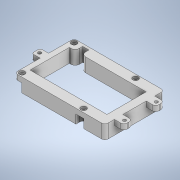
# Autodesk Inventor part: Pi3BatteryBoard_Mockup
Saved by Autodesk Inventor 2021 (Build 250183000, 183)
## iProperties
Created: 2021-04-19
Part Number: Pi3BatteryBoard_Mockup
Material: Generic
Document SubType Name: Modeling
Designer: trent
Density: 1 g/cm^3
Appearance: Default
Author: trent
Autodesk Inventor part; units mm, degrees
ref_plane "YZ Plane" through (0, 0, 0) normal (1, 0, 0) x (0, 1, 0)
ref_plane "XZ Plane" through (0, 0, 0) normal (0, 1, 0) x (-1, 0, 0)
ref_plane "XY Plane" through (0, 0, 0) normal (0, 0, 1) x (1, 0, 0)
sketch "Sketch1" plane through (0, 0, 0) normal (0, 1, 0) x (-1, 0, 0)
  line L0 (-3, 0) -> (-82, 0)
  line L1 (-85, -3) -> (-85, -53)
  line L2 (-82, -56) -> (-3, -56)
  line L3 (0, -53) -> (0, -3)
  arc A0 (-3, -56) -> (0, -53) centre (-3, -53) ccw
  arc A1 (0, -3) -> (-3, 0) centre (-3, -3) ccw
  arc A2 (-82, 0) -> (-85, -3) centre (-82, -3) ccw
  arc A3 (-85, -53) -> (-82, -56) centre (-82, -53) ccw
  circle A4 centre (-3.5, -52.5) radius 1.5
  circle A5 centre (-3.5, -3.5) radius 1.5
  circle A6 centre (-61.5, -52.5) radius 1.5
  circle A7 centre (-61.5, -3.5) radius 1.5
  point P0 (0, 0)
  point P1 (-85, -56)
  point P2 (-85, 0)
  point P3 (0, -56)
  dimension "d0" = 85
  dimension "d1" = 56
  dimension "d2" = 3
  dimension "d9" = 3
  dimension "d10" = 3
  dimension "d15" = 3
  dimension "d16" = 3
  dimension "d140" = 58
  dimension "d141" = 58
  dimension "d142" = 49
  dimension "d143" = 3.5
  constraints: 8 centre point, 8 end point, 8 point on circle, 8 point on line, 8 tangent, 3 equal radius, 2 parallel, 1 horizontal, 1 perpendicular
  measures "d0" distance of point (-85, -56) point (0, -56)
  measures "d1" distance of point (-85, 0) point (-85, -56)
  measures "d2" radius of A0
  measures "d9" diameter of A4
  measures "d10" diameter of A5
  measures "d15" diameter of A6
  measures "d16" diameter of A7
  measures "d140" distance of A6.centre A4.centre
  measures "d141" distance of A5.centre A7.centre
  measures "d142" distance of A4.centre A5.centre
  measures "d143" distance from line of L0 A5.centre
extrude "Extrusion1" add sketch "Sketch1" along normal blind 13
sketch "Sketch12" plane through (0, 0, 0) normal (0, -1, 0) x (1, 0, 0)
  line L0 (5, -9.5) -> (77.5, -9.5)
  line L1 (77.5, -9.5) -> (77.5, -46.5)
  line L2 (5, -46.5) -> (5, -9.5)
  line L3 (82, -56) -> (3, -56) projected
  line L4 (85, -3) -> (85, -53) projected
  line L5 (3, 0) -> (82, 0) projected
  line L6 (0, -53) -> (0, -3) projected
  line L7 (16.35, -50.5) -> (16.35, -53.65)
  line L8 (16.35, -53.65) -> (10.5, -53.65)
  line L9 (10.5, -53.65) -> (10.5, -50.5)
  line L10 (77.5, -46.5) -> (20.35, -46.5)
  line L11 (6.5, -46.5) -> (5, -46.5)
  arc A0 (10.5, -50.5) -> (6.5, -46.5) centre (6.5, -50.5) ccw
  arc A1 (20.35, -46.5) -> (16.35, -50.5) centre (20.35, -50.5) ccw
  point P0 (0, 0)
  point P1 (10.5, -46.5)
  point P2 (16.35, -46.5)
  dimension "d153" = 7.5
  dimension "d154" = 9.5
  dimension "d155" = 5
  dimension "d157" = 10.5
  dimension "d158" = 2.35
  dimension "d159" = 5.85
  dimension "d160" = 4
  constraints: 16 end point, 4 parallel, 4 point on circle, 4 point on line, 4 tangent, 2 centre point, 1 equal radius, 1 horizontal, 1 perpendicular
  measures "d153" distance between parallel lines of L4 L1
  measures "d154" distance between parallel lines of L5 L0
  measures "d155" distance between parallel lines of L6 L2
  measures "d157" distance between parallel lines of L6 L9
  measures "d158" distance between parallel lines of L3 L8
  measures "d159" distance of L7.end L8.end
  measures "d160" radius of A0
extrude "Extrusion12" cut sketch "Sketch12" against normal up to next
sketch "Sketch14" plane through (0, 13, 0) normal (0, 1, 0) x (1, 0, 0)
  circle A0 centre (3.5, 3.5) radius 1.5 projected
  circle A1 centre (3.5, 3.5) radius 2.625
  circle A2 centre (61.5, 3.5) radius 1.5 projected
  circle A3 centre (61.5, 3.5) radius 2.625
  circle A4 centre (61.5, 52.5) radius 1.5 projected
  circle A5 centre (61.5, 52.5) radius 2.625
  circle A6 centre (3.5, 52.5) radius 1.5 projected
  circle A7 centre (3.5, 52.5) radius 2.625
  point P0 (0, 0)
  dimension "d161" = 5.25
  dimension "d162" = 5.25
  dimension "d163" = 5.25
  dimension "d164" = 5.25
  constraints: 4 centre point, 4 coincident
  measures "d161" diameter of A1
  measures "d162" diameter of A7
  measures "d163" diameter of A5
  measures "d164" diameter of A3
extrude "Extrusion14" cut sketch "Sketch14" against normal blind 1.75 contours A0 | A1 | A2 | A3 | A4 | A5 | A6 | A7
sketch "Sketch15" plane through (0, 0, 0) normal (0, -1, 0) x (1, 0, 0)
  arc A0 (3.5, -6.75) -> (6.75, -3.5) centre (3.5, -3.5) ccw
  arc A1 (57.75, -3.5) -> (65.25, -3.5) centre (61.5, -3.5) ccw
  arc A2 (65.25, -52.5) -> (57.75, -52.5) centre (61.5, -52.5) ccw
  arc A3 (6.75, -52.5) -> (3.5, -49.25) centre (3.5, -52.5) ccw
  line L0 (57.75, -3.5) -> (57.75, 0)
  line L1 (3, 0) -> (82, 0) projected
  line L2 (65.25, -3.5) -> (65.25, 0)
  line L3 (65.25, -52.5) -> (65.25, -56)
  line L4 (82, -56) -> (3, -56) projected
  line L5 (57.75, -52.5) -> (57.75, -56)
  line L6 (6.75, -3.5) -> (6.75, 0)
  line L7 (3.5, -6.75) -> (0, -6.75)
  line L8 (0, -53) -> (0, -3) projected
  line L9 (3.5, -49.25) -> (0, -49.25)
  line L10 (6.75, -52.5) -> (6.75, -56)
  line L11 (65.25, 0) -> (57.75, 0)
  line L12 (65.25, -56) -> (57.75, -56)
  arc A4 (0, -53) -> (3, -56) centre (3, -53) ccw projected
  line L13 (6.75, -56) -> (3, -56)
  line L14 (0, -49.25) -> (0, -53)
  line L15 (0, -6.75) -> (0, -3)
  line L16 (3, 0) -> (6.75, 0)
  arc A5 (3, 0) -> (0, -3) centre (3, -3) ccw projected
  arc A6 (3, 0) -> (0, -3) centre (3, -3) ccw
  arc A7 (0, -53) -> (3, -56) centre (3, -53) ccw
  point P0 (0, 0)
  dimension "d167" = 6.5
  dimension "d168" = 6.5
  dimension "d169" = 7.5
  dimension "d170" = 7.5
  constraints: 29 end point, 13 point on circle, 9 point on line, 7 tangent, 6 centre point, 6 coincident, 4 collinear, 4 vertical, 3 horizontal, 3 perpendicular, 1 concentric
  measures "d167" diameter of A0
  measures "d168" diameter of A3
  measures "d169" diameter of A2
  measures "d170" diameter of A1
extrude "Extrusion15" cut sketch "Sketch15" against normal blind 8.25
sketch "Sketch16" plane through (0, 13, 0) normal (0, 1, 0) x (1, 0, 0)
  line L0 (5, 9.5) -> (5, 46.5) projected
  line L1 (0, 49.25) -> (0, 6.75) projected
  line L2 (0, 32) -> (-6, 32)
  line L3 (-8, 30) -> (-8, 26)
  line L4 (-6, 24) -> (0, 24)
  line L5 (0, 24) -> (0, 32)
  circle A0 centre (-4.5, 28) radius 1.5
  arc A1 (-6, 32) -> (-8, 30) centre (-6, 30) ccw
  arc A2 (-8, 26) -> (-6, 24) centre (-6, 26) ccw
  line L6 (3, 0) -> (82, 0) projected
  line L7 (42.5, 0) -> (42.5, 9.5)
  line L8 (85, 39) -> (90.6651, 39)
  line L9 (94, 42.3349) -> (94, 43.6651)
  line L10 (90.6651, 47) -> (85, 47)
  line L11 (85, 47) -> (85, 39)
  circle A3 centre (90.5, 43) radius 1.5
  arc A4 (90.6651, 39) -> (94, 42.3349) centre (90.6651, 42.3349) ccw
  arc A5 (94, 43.6651) -> (90.6651, 47) centre (90.6651, 43.6651) ccw
  line L12 (85, 3) -> (85, 53) projected
  line L13 (82, 56) -> (3, 56) projected
  line L14 (85, 17) -> (85, 9)
  line L15 (90.6651, 17) -> (85, 17)
  line L16 (85, 9) -> (90.6651, 9)
  circle A6 centre (90.5, 13) radius 1.5
  arc A7 (94, 13.6651) -> (90.6651, 17) centre (90.6651, 13.6651) ccw
  line L17 (94, 12.3349) -> (94, 13.6651)
  arc A8 (90.6651, 9) -> (94, 12.3349) centre (90.6651, 12.3349) ccw
  point P0 (0, 0)
  point P1 (0, 28)
  point P2 (-8, 24)
  point P3 (-8, 32)
  point P4 (94, 47)
  point P5 (94, 39)
  point P6 (85, 28)
  point P7 (94, 17)
  point P8 (94, 9)
  point P9 (0, 24)
  dimension "d175" = 4
  dimension "d176" = 8
  dimension "d177" = 8
  dimension "d178" = 4
  dimension "d179" = 3.5
  dimension "d180" = 2
  dimension "d183" = 8
  dimension "d184" = 9
  dimension "d185" = 4
  dimension "d186" = 3.5
  dimension "d188" = 0
  dimension "d189" = 9
  dimension "d190" = 8
  dimension "d191" = 9
  dimension "d192" = 4
  dimension "d193" = 3.5
  dimension "d194" = 9
  dimension "d197" = 3
  dimension "d198" = 3
  dimension "d199" = 3
  dimension "d200" = 24
  constraints: 26 end point, 13 point on line, 12 point on circle, 12 tangent, 9 centre point, 6 parallel, 3 equal radius, 3 midpoint, 3 perpendicular, 1 horizontal, 1 vertical
  measures "d175" distance from line of point (0, 28) L2
  measures "d176" distance of point (-8, 32) point (-8, 24)
  measures "d177" distance of L2.start point (-8, 32)
  measures "d178" distance from line of L2 A0.centre
  measures "d179" distance from line of L3 A0.centre
  measures "d180" radius of A1
  measures "d183" distance of point (94, 39) point (94, 47)
  measures "d184" distance of L11.end point (94, 39)
  measures "d185" distance from line of L8 A3.centre
  measures "d186" distance from line of L9 A3.centre
  measures "d188" distance between parallel lines of L12 L11
  measures "d189" distance between parallel lines of L13 L10
  measures "d190" distance of point (94, 9) point (94, 17)
  measures "d191" distance of L14.end point (94, 9)
  measures "d192" distance from line of L16 A6.centre
  measures "d193" distance from line of L17 A6.centre
  measures "d194" distance between parallel lines of L6 L16
  measures "d197" diameter of A0
  measures "d198" diameter of A3
  measures "d199" diameter of A6
  measures "d200" distance between parallel lines of L6 L4
extrude "Extrusion16" add sketch "Sketch16" against normal blind 5
equation "\"d10\" = d9"
equation "\"d15\" = d9"
equation "\"d16\" = d9"
equation "\"d162\" = d161"
equation "\"d163\" = d161"
equation "\"d164\" = d161"
equation "\"d175\" = 0.5 * d176"
equation "\"d178\" = d175"
equation "\"d185\" = 0.5 * d183"
equation "\"d192\" = 0.5 * d190"
equation "\"d198\" = d197"
equation "\"d199\" = d197"
equation "\"d182\" = 0.5 * d183"
body "Solid1"
